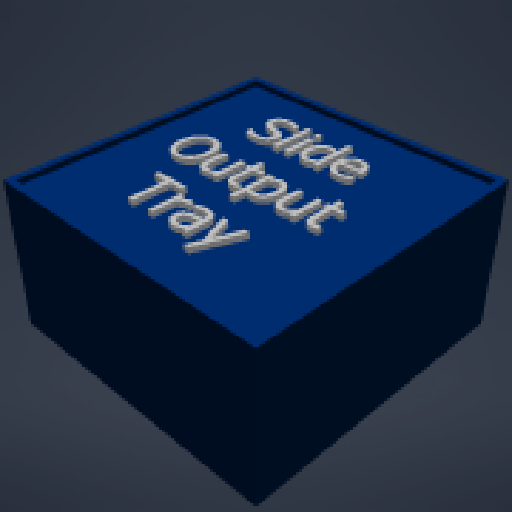
# Autodesk Inventor part: Slide Export Tray
Saved by Autodesk Inventor 2025.1 (Build 291241000, 241)
## iProperties
Created: 2024-10-31
Part Number: Slide Export Tray
Material: Generic
Document SubType Name: Modeling
Designer: jerem
Density: 1 g/cm^3
Appearance: Default
Author: jerem
Autodesk Inventor part; units mm, degrees
ref_plane "YZ Plane" through (0, 0, 0) normal (1, 0, 0) x (0, 1, 0)
ref_plane "XZ Plane" through (0, 0, 0) normal (0, 1, 0) x (-1, 0, 0)
ref_plane "XY Plane" through (0, 0, 0) normal (0, 0, 1) x (1, 0, 0)
sketch "Sketch1" plane through (0, 0, 0) normal (0, 1, 0) x (-1, 0, 0)
  line L0 (-50, 50) -> (50, 50)
  line L1 (50, 50) -> (50, -50)
  line L2 (50, -50) -> (-50, -50)
  line L3 (-50, -50) -> (-50, 50)
  line L4 (-50, 50) -> (50, -50) construction
  line L5 (50, 50) -> (-50, -50) construction
  line L6 (-47.5, 47.5) -> (47.5, 47.5)
  line L7 (47.5, 47.5) -> (47.5, -47.5)
  line L8 (47.5, -47.5) -> (-47.5, -47.5)
  line L9 (-47.5, -47.5) -> (-47.5, 47.5)
  line L10 (-47.5, 47.5) -> (47.5, -47.5) construction
  line L11 (47.5, 47.5) -> (-47.5, -47.5) construction
  point P0 (0, 0)
  dimension "d0" = 100
  dimension "d1" = 100
  dimension "d3" = 95
  constraints: 24 end point, 4 midpoint, 4 parallel, 2 horizontal, 2 perpendicular, 1 point on line
  measures "d0" distance of L1.end L2.end
  measures "d1" distance of L0.end L1.end
  measures "d3" distance of L7.end L8.end
extrude "Extrusion1" add sketch "Sketch1" along normal blind 50 contours L0 L1 L2 L3 | L6 L7 L8 L9
extrude "Extrusion2" add sketch "Sketch1" along normal blind 2 from surface at 50
sketch "Sketch2" plane through (0, 50, 0) normal (0, 1, 0) x (1, 0, 0)
  line L0 (-37.0883, 25.1556) -> (31.9282, 25.1556) construction
  line L1 (31.9282, 25.1556) -> (31.9282, -26.4456) construction
  line L2 (31.9282, -26.4456) -> (-37.0883, -26.4456) construction
  line L3 (-37.0883, -26.4456) -> (-37.0883, 25.1556) construction
  spline S0 degree 2 poles (-18.4674, 18.0229) (-20.0963, 18.0229) (-22.3815, 18.7036) (-23.3904, 19.1899) knots 0 0 0 1 2 2 2
  line L4 (-23.3904, 19.1899) -> (-23.3904, 21.6939)
  line L5 (-23.3904, 21.6939) -> (-23.2446, 21.6939)
  spline S1 degree 2 poles (-23.2446, 21.6939) (-22.26, 20.7701) (-19.7681, 19.749) (-18.6133, 19.749) knots 0 0 0 1 2 2 2
  spline S2 degree 2 poles (-18.6133, 19.749) (-16.9601, 19.749) (-15.2705, 21.1226) (-15.2705, 22.2531) knots 0 0 0 1 2 2 2
  spline S3 degree 2 poles (-15.2705, 22.2531) (-15.2705, 23.1526) (-16.1579, 24.2709) (-17.1181, 24.5505) knots 0 0 0 1 2 2 2
  spline S4 degree 2 poles (-17.1181, 24.5505) (-17.811, 24.745) (-18.9658, 25.0124) (-19.8288, 25.2312) knots 0 0 0 1 2 2 2
  spline S5 degree 2 poles (-19.8288, 25.2312) (-20.6068, 25.4378) (-21.8345, 26.0578) (-22.3086, 26.5561) knots 0 0 0 1 2 2 2
  spline S6 degree 2 poles (-22.3086, 26.5561) (-22.7705, 27.0545) (-23.281, 28.3916) (-23.281, 29.2668) knots 0 0 0 1 2 2 2
  spline S7 degree 2 poles (-23.281, 29.2668) (-23.281, 31.0902) (-20.4366, 33.5578) (-18.2365, 33.5578) knots 0 0 0 1 2 2 2
  spline S8 degree 2 poles (-18.2365, 33.5578) (-16.9723, 33.5578) (-14.7356, 33.0594) (-13.7754, 32.5853) knots 0 0 0 1 2 2 2
  line L6 (-13.7754, 32.5853) -> (-13.7754, 30.2028)
  line L7 (-13.7754, 30.2028) -> (-13.9212, 30.2028)
  spline S9 degree 2 poles (-13.9212, 30.2028) (-14.6384, 30.8592) (-16.875, 31.8317) (-18.1027, 31.8317) knots 0 0 0 1 2 2 2
  spline S10 degree 2 poles (-18.1027, 31.8317) (-19.4885, 31.8317) (-21.2024, 30.531) (-21.2024, 29.4735) knots 0 0 0 1 2 2 2
  spline S11 degree 2 poles (-21.2024, 29.4735) (-21.2024, 28.5253) (-20.1935, 27.3949) (-19.2454, 27.1396) knots 0 0 0 1 2 2 2
  spline S12 degree 2 poles (-19.2454, 27.1396) (-18.6133, 26.9694) (-16.7778, 26.5318) (-16.17, 26.3495) knots 0 0 0 1 2 2 2
  spline S13 degree 2 poles (-16.17, 26.3495) (-14.6262, 25.8754) (-13.1919, 23.967) (-13.1919, 22.5691) knots 0 0 0 1 2 2 2
  spline S14 degree 2 poles (-13.1919, 22.5691) (-13.1919, 21.6818) (-13.9091, 19.98) (-14.5533, 19.3843) knots 0 0 0 1 2 2 2
  spline S15 degree 2 poles (-14.5533, 19.3843) (-15.2705, 18.7279) (-17.0938, 18.0229) (-18.4674, 18.0229) knots 0 0 0 1 2 2 2
  line L8 (-9.375, 18.2903) -> (-11.2713, 18.2903)
  line L9 (-11.2713, 18.2903) -> (-11.2713, 33.9589)
  line L10 (-11.2713, 33.9589) -> (-9.375, 33.9589)
  line L11 (-9.375, 33.9589) -> (-9.375, 18.2903)
  line L12 (-4.6587, 18.2903) -> (-6.5549, 18.2903)
  line L13 (-6.5549, 18.2903) -> (-6.5549, 29.5464)
  line L14 (-6.5549, 29.5464) -> (-4.6587, 29.5464)
  line L15 (-4.6587, 29.5464) -> (-4.6587, 18.2903)
  line L16 (-4.525, 31.4184) -> (-6.6765, 31.4184)
  line L17 (-6.6765, 31.4184) -> (-6.6765, 33.3876)
  line L18 (-6.6765, 33.3876) -> (-4.525, 33.3876)
  line L19 (-4.525, 33.3876) -> (-4.525, 31.4184)
  line L20 (6.7797, 18.2903) -> (4.8835, 18.2903)
  line L21 (4.8835, 18.2903) -> (4.8835, 19.433)
  spline S16 degree 2 poles (4.8835, 19.433) (4.4459, 19.0683) (3.8016, 18.5821) (3.364, 18.3754) knots 0 0 0 1 2 2 2
  spline S17 degree 2 poles (3.364, 18.3754) (2.9629, 18.1809) (2.0998, 17.9743) (1.5285, 17.9743) knots 0 0 0 1 2 2 2
  spline S18 degree 2 poles (1.5285, 17.9743) (0.6047, 17.9743) (-0.9512, 18.7401) (-1.4982, 19.4816) knots 0 0 0 1 2 2 2
  spline S19 degree 2 poles (-1.4982, 19.4816) (-2.0452, 20.2231) (-2.653, 22.4111) (-2.653, 23.8333) knots 0 0 0 1 2 2 2
  spline S20 degree 2 poles (-2.653, 23.8333) (-2.653, 25.3163) (-1.8872, 27.48) (-1.2186, 28.2944) knots 0 0 0 1 2 2 2
  spline S21 degree 2 poles (-1.2186, 28.2944) (-0.5987, 29.0237) (1.1396, 29.8625) (2.0998, 29.8625) knots 0 0 0 1 2 2 2
  spline S22 degree 2 poles (2.0998, 29.8625) (2.9386, 29.8625) (4.1906, 29.4856) (4.8835, 29.0967) knots 0 0 0 1 2 2 2
  line L22 (4.8835, 29.0967) -> (4.8835, 33.9589)
  line L23 (4.8835, 33.9589) -> (6.7797, 33.9589)
  line L24 (6.7797, 33.9589) -> (6.7797, 18.2903)
  line L25 (4.8835, 21.0253) -> (4.8835, 27.5286)
  spline S23 degree 2 poles (4.8835, 27.5286) (4.1785, 27.8689) (3.0601, 28.1242) (2.4159, 28.1242) knots 0 0 0 1 2 2 2
  spline S24 degree 2 poles (2.4159, 28.1242) (0.9572, 28.1242) (-0.6959, 25.9362) (-0.6959, 23.8698) knots 0 0 0 1 2 2 2
  spline S25 degree 2 poles (-0.6959, 23.8698) (-0.6959, 21.8762) (0.5682, 19.7733) (1.9661, 19.7733) knots 0 0 0 1 2 2 2
  spline S26 degree 2 poles (1.9661, 19.7733) (2.7076, 19.7733) (4.2149, 20.454) (4.8835, 21.0253) knots 0 0 0 1 2 2 2
  spline S27 degree 2 poles (14.4135, 18.0351) (11.7149, 18.0351) (8.749, 21.0618) (8.749, 23.8576) knots 0 0 0 1 2 2 2
  spline S28 degree 2 poles (8.749, 23.8576) (8.749, 26.6048) (11.6298, 29.8625) (13.9515, 29.8625) knots 0 0 0 1 2 2 2
  spline S29 degree 2 poles (13.9515, 29.8625) (14.9969, 29.8625) (16.6136, 29.2547) (17.2092, 28.6104) knots 0 0 0 1 2 2 2
  spline S30 degree 2 poles (17.2092, 28.6104) (17.817, 27.9662) (18.4613, 26.1064) (18.4613, 24.7571) knots 0 0 0 1 2 2 2
  line L26 (18.4613, 24.7571) -> (18.4613, 23.7239)
  line L27 (18.4613, 23.7239) -> (10.6695, 23.7239)
  spline S31 degree 2 poles (10.6695, 23.7239) (10.6695, 21.7668) (12.6387, 19.6882) (14.3891, 19.6882) knots 0 0 0 1 2 2 2
  spline S32 degree 2 poles (14.3891, 19.6882) (15.0091, 19.6882) (16.2125, 19.9678) (16.6987, 20.1866) knots 0 0 0 1 2 2 2
  spline S33 degree 2 poles (16.6987, 20.1866) (17.2092, 20.4297) (17.9143, 20.8552) (18.1452, 21.0497) knots 0 0 0 1 2 2 2
  line L28 (18.1452, 21.0497) -> (18.2546, 21.0497)
  line L29 (18.2546, 21.0497) -> (18.2546, 18.9832)
  spline S34 degree 2 poles (18.2546, 18.9832) (17.9264, 18.8495) (16.9297, 18.4605) (16.5407, 18.3511) knots 0 0 0 1 2 2 2
  spline S35 degree 2 poles (16.5407, 18.3511) (15.9937, 18.1931) (15.0942, 18.0351) (14.4135, 18.0351) knots 0 0 0 1 2 2 2
  spline S36 degree 2 poles (16.6136, 25.1704) (16.5893, 25.9362) (16.2733, 27.0545) (15.9694, 27.4313) knots 0 0 0 1 2 2 2
  spline S37 degree 2 poles (15.9694, 27.4313) (15.6412, 27.8568) (14.6079, 28.3065) (13.8421, 28.3065) knots 0 0 0 1 2 2 2
  spline S38 degree 2 poles (13.8421, 28.3065) (13.0885, 28.3065) (12.031, 27.8568) (11.5934, 27.4192) knots 0 0 0 1 2 2 2
  spline S39 degree 2 poles (11.5934, 27.4192) (11.1679, 26.9694) (10.7303, 25.8876) (10.6695, 25.1704) knots 0 0 0 1 2 2 2
  line L30 (10.6695, 25.1704) -> (16.6136, 25.1704)
  spline S40 degree 2 poles (-21.8527, 6.8793) (-21.0019, 5.8825) (-20.0537, 2.9652) (-20.0537, 1.0932) knots 0 0 0 1 2 2 2
  spline S41 degree 2 poles (-20.0537, 1.0932) (-20.0537, -0.7301) (-20.9775, -3.6839) (-21.8527, -4.6807) knots 0 0 0 1 2 2 2
  spline S42 degree 2 poles (-21.8527, -4.6807) (-22.7766, -5.7261) (-25.2198, -6.7228) (-26.6907, -6.7228) knots 0 0 0 1 2 2 2
  spline S43 degree 2 poles (-26.6907, -6.7228) (-28.2101, -6.7228) (-30.6412, -5.6896) (-31.5286, -4.6807) knots 0 0 0 1 2 2 2
  spline S44 degree 2 poles (-31.5286, -4.6807) (-32.3916, -3.6839) (-33.3155, -0.7544) (-33.3155, 1.0932) knots 0 0 0 1 2 2 2
  spline S45 degree 2 poles (-33.3155, 1.0932) (-33.3155, 2.9774) (-32.3795, 5.8461) (-31.5164, 6.8793) knots 0 0 0 1 2 2 2
  spline S46 degree 2 poles (-31.5164, 6.8793) (-30.6412, 7.8761) (-28.198, 8.9093) (-26.6907, 8.9093) knots 0 0 0 1 2 2 2
  spline S47 degree 2 poles (-26.6907, 8.9093) (-25.1591, 8.9093) (-22.7036, 7.8396) (-21.8527, 6.8793) knots 0 0 0 1 2 2 2
  spline S48 degree 2 poles (-22.1323, 1.0932) (-22.1323, 2.5762) (-22.7766, 4.8736) (-23.36, 5.6273) knots 0 0 0 1 2 2 2
  spline S49 degree 2 poles (-23.36, 5.6273) (-23.9557, 6.4052) (-25.6331, 7.1832) (-26.6785, 7.1832) knots 0 0 0 1 2 2 2
  spline S50 degree 2 poles (-26.6785, 7.1832) (-27.7604, 7.1832) (-29.3892, 6.4295) (-30.0091, 5.6273) knots 0 0 0 1 2 2 2
  spline S51 degree 2 poles (-30.0091, 5.6273) (-30.6048, 4.8615) (-31.2369, 2.5519) (-31.2369, 1.0932) knots 0 0 0 1 2 2 2
  spline S52 degree 2 poles (-31.2369, 1.0932) (-31.2369, -1.8606) (-28.7571, -4.9967) (-26.6785, -4.9967) knots 0 0 0 1 2 2 2
  spline S53 degree 2 poles (-26.6785, -4.9967) (-24.5999, -4.9967) (-22.1323, -1.8606) (-22.1323, 1.0932) knots 0 0 0 1 2 2 2
  line L31 (-9.2596, -6.4068) -> (-11.1558, -6.4068)
  line L32 (-11.1558, -6.4068) -> (-11.1558, -5.1669)
  spline S54 degree 2 poles (-11.1558, -5.1669) (-12.031, -5.9327) (-13.5991, -6.7228) (-14.5715, -6.7228) knots 0 0 0 1 2 2 2
  spline S55 degree 2 poles (-14.5715, -6.7228) (-15.3009, -6.7228) (-16.6015, -6.2366) (-17.0756, -5.7139) knots 0 0 0 1 2 2 2
  spline S56 degree 2 poles (-17.0756, -5.7139) (-17.5618, -5.1912) (-18.0967, -3.5988) (-18.0967, -2.4562) knots 0 0 0 1 2 2 2
  line L33 (-18.0967, -2.4562) -> (-18.0967, 4.8493)
  line L34 (-18.0967, 4.8493) -> (-16.2004, 4.8493)
  line L35 (-16.2004, 4.8493) -> (-16.2004, -1.5688)
  spline S57 degree 2 poles (-16.2004, -1.5688) (-16.2004, -2.4684) (-16.0667, -3.6474) (-15.8357, -4.085) knots 0 0 0 1 2 2 2
  spline S58 degree 2 poles (-15.8357, -4.085) (-15.6048, -4.5226) (-14.8147, -4.9238) (-14.0732, -4.9238) knots 0 0 0 1 2 2 2
  spline S59 degree 2 poles (-14.0732, -4.9238) (-13.3803, -4.9238) (-11.8122, -4.1337) (-11.1558, -3.5624) knots 0 0 0 1 2 2 2
  line L36 (-11.1558, -3.5624) -> (-11.1558, 4.8493)
  line L37 (-11.1558, 4.8493) -> (-9.2596, 4.8493)
  line L38 (-9.2596, 4.8493) -> (-9.2596, -6.4068)
  spline S60 degree 2 poles (-3.1088, -6.6256) (-4.6526, -6.6256) (-6.3908, -4.863) (-6.3908, -2.9546) knots 0 0 0 1 2 2 2
  line L39 (-6.3908, -2.9546) -> (-6.3908, 3.2812)
  line L40 (-6.3908, 3.2812) -> (-7.6672, 3.2812)
  line L41 (-7.6672, 3.2812) -> (-7.6672, 4.8493)
  line L42 (-7.6672, 4.8493) -> (-6.3908, 4.8493)
  line L43 (-6.3908, 4.8493) -> (-6.3908, 8.0827)
  line L44 (-6.3908, 8.0827) -> (-4.4946, 8.0827)
  line L45 (-4.4946, 8.0827) -> (-4.4946, 4.8493)
  line L46 (-4.4946, 4.8493) -> (-1.0059, 4.8493)
  line L47 (-1.0059, 4.8493) -> (-1.0059, 3.2812)
  line L48 (-1.0059, 3.2812) -> (-4.4946, 3.2812)
  line L49 (-4.4946, 3.2812) -> (-4.4946, -2.0794)
  spline S61 degree 2 poles (-4.4946, -2.0794) (-4.4946, -2.9303) (-4.4338, -3.8662) (-4.2271, -4.2674) knots 0 0 0 1 2 2 2
  spline S62 degree 2 poles (-4.2271, -4.2674) (-4.057, -4.6199) (-3.2912, -4.9724) (-2.6348, -4.9724) knots 0 0 0 1 2 2 2
  spline S63 degree 2 poles (-2.6348, -4.9724) (-2.1728, -4.9724) (-1.3098, -4.6928) (-1.1153, -4.6077) knots 0 0 0 1 2 2 2
  line L50 (-1.1153, -4.6077) -> (-1.0059, -4.6077)
  line L51 (-1.0059, -4.6077) -> (-1.0059, -6.3095)
  spline S64 degree 2 poles (-1.0059, -6.3095) (-1.5408, -6.4554) (-2.6348, -6.6256) (-3.1088, -6.6256) knots 0 0 0 1 2 2 2
  spline S65 degree 2 poles (9.8247, -0.4748) (9.8247, -3.2949) (7.1383, -6.6256) (5.084, -6.6256) knots 0 0 0 1 2 2 2
  spline S66 degree 2 poles (5.084, -6.6256) (4.2453, -6.6256) (2.9568, -6.2366) (2.2883, -5.8355) knots 0 0 0 1 2 2 2
  line L52 (2.2883, -5.8355) -> (2.2883, -10.5518)
  line L53 (2.2883, -10.5518) -> (0.392, -10.5518)
  line L54 (0.392, -10.5518) -> (0.392, 4.8493)
  line L55 (0.392, 4.8493) -> (2.2883, 4.8493)
  line L56 (2.2883, 4.8493) -> (2.2883, 3.6702)
  spline S67 degree 2 poles (2.2883, 3.6702) (2.9933, 4.3145) (4.7194, 5.1654) (5.7283, 5.1654) knots 0 0 0 1 2 2 2
  spline S68 degree 2 poles (5.7283, 5.1654) (7.661, 5.1654) (9.8247, 2.1021) (9.8247, -0.4748) knots 0 0 0 1 2 2 2
  spline S69 degree 2 poles (7.8677, -0.6936) (7.8677, 1.2391) (6.64, 3.3663) (5.2664, 3.3663) knots 0 0 0 1 2 2 2
  spline S70 degree 2 poles (5.2664, 3.3663) (4.4641, 3.3663) (2.9568, 2.6492) (2.2883, 2.09) knots 0 0 0 1 2 2 2
  line L57 (2.2883, 2.09) -> (2.2883, -4.3038)
  spline S71 degree 2 poles (2.2883, -4.3038) (3.0297, -4.6564) (4.0873, -4.9238) (4.768, -4.9238) knots 0 0 0 1 2 2 2
  spline S72 degree 2 poles (4.768, -4.9238) (6.2388, -4.9238) (7.8677, -2.7601) (7.8677, -0.6936) knots 0 0 0 1 2 2 2
  line L58 (20.546, -6.4068) -> (18.6497, -6.4068)
  line L59 (18.6497, -6.4068) -> (18.6497, -5.1669)
  spline S73 degree 2 poles (18.6497, -5.1669) (17.7745, -5.9327) (16.2064, -6.7228) (15.234, -6.7228) knots 0 0 0 1 2 2 2
  spline S74 degree 2 poles (15.234, -6.7228) (14.5046, -6.7228) (13.204, -6.2366) (12.7299, -5.7139) knots 0 0 0 1 2 2 2
  spline S75 degree 2 poles (12.7299, -5.7139) (12.2437, -5.1912) (11.7088, -3.5988) (11.7088, -2.4562) knots 0 0 0 1 2 2 2
  line L60 (11.7088, -2.4562) -> (11.7088, 4.8493)
  line L61 (11.7088, 4.8493) -> (13.6051, 4.8493)
  line L62 (13.6051, 4.8493) -> (13.6051, -1.5688)
  spline S76 degree 2 poles (13.6051, -1.5688) (13.6051, -2.4684) (13.7388, -3.6474) (13.9698, -4.085) knots 0 0 0 1 2 2 2
  spline S77 degree 2 poles (13.9698, -4.085) (14.2007, -4.5226) (14.9909, -4.9238) (15.7323, -4.9238) knots 0 0 0 1 2 2 2
  spline S78 degree 2 poles (15.7323, -4.9238) (16.4252, -4.9238) (17.9933, -4.1337) (18.6497, -3.5624) knots 0 0 0 1 2 2 2
  line L63 (18.6497, -3.5624) -> (18.6497, 4.8493)
  line L64 (18.6497, 4.8493) -> (20.546, 4.8493)
  line L65 (20.546, 4.8493) -> (20.546, -6.4068)
  spline S79 degree 2 poles (26.6967, -6.6256) (25.1529, -6.6256) (23.4147, -4.863) (23.4147, -2.9546) knots 0 0 0 1 2 2 2
  line L66 (23.4147, -2.9546) -> (23.4147, 3.2812)
  line L67 (23.4147, 3.2812) -> (22.1383, 3.2812)
  line L68 (22.1383, 3.2812) -> (22.1383, 4.8493)
  line L69 (22.1383, 4.8493) -> (23.4147, 4.8493)
  line L70 (23.4147, 4.8493) -> (23.4147, 8.0827)
  line L71 (23.4147, 8.0827) -> (25.3109, 8.0827)
  line L72 (25.3109, 8.0827) -> (25.3109, 4.8493)
  line L73 (25.3109, 4.8493) -> (28.7996, 4.8493)
  line L74 (28.7996, 4.8493) -> (28.7996, 3.2812)
  line L75 (28.7996, 3.2812) -> (25.3109, 3.2812)
  line L76 (25.3109, 3.2812) -> (25.3109, -2.0794)
  spline S80 degree 2 poles (25.3109, -2.0794) (25.3109, -2.9303) (25.3717, -3.8662) (25.5784, -4.2674) knots 0 0 0 1 2 2 2
  spline S81 degree 2 poles (25.5784, -4.2674) (25.7485, -4.6199) (26.5144, -4.9724) (27.1708, -4.9724) knots 0 0 0 1 2 2 2
  spline S82 degree 2 poles (27.1708, -4.9724) (27.6327, -4.9724) (28.4957, -4.6928) (28.6902, -4.6077) knots 0 0 0 1 2 2 2
  line L77 (28.6902, -4.6077) -> (28.7996, -4.6077)
  line L78 (28.7996, -4.6077) -> (28.7996, -6.3095)
  spline S83 degree 2 poles (28.7996, -6.3095) (28.2648, -6.4554) (27.1708, -6.6256) (26.6967, -6.6256) knots 0 0 0 1 2 2 2
  line L79 (-17.8536, -31.1039) -> (-17.8536, -17.8786)
  line L80 (-17.8536, -17.8786) -> (-22.886, -17.8786)
  line L81 (-22.886, -17.8786) -> (-22.886, -16.1039)
  line L82 (-22.886, -16.1039) -> (-10.8276, -16.1039)
  line L83 (-10.8276, -16.1039) -> (-10.8276, -17.8786)
  line L84 (-10.8276, -17.8786) -> (-15.86, -17.8786)
  line L85 (-15.86, -17.8786) -> (-15.86, -31.1039)
  line L86 (-15.86, -31.1039) -> (-17.8536, -31.1039)
  line L87 (-3.4856, -21.8778) -> (-3.5829, -21.8778)
  spline S84 degree 2 poles (-3.5829, -21.8778) (-3.8017, -21.817) (-4.2758, -21.7927) (-4.604, -21.7927) knots 0 0 0 1 2 2 2
  spline S85 degree 2 poles (-4.604, -21.7927) (-5.3698, -21.7927) (-6.8771, -22.4612) (-7.5578, -23.1176) knots 0 0 0 1 2 2 2
  line L88 (-7.5578, -23.1176) -> (-7.5578, -31.1039)
  line L89 (-7.5578, -31.1039) -> (-9.454, -31.1039)
  line L90 (-9.454, -31.1039) -> (-9.454, -19.8478)
  line L91 (-9.454, -19.8478) -> (-7.5578, -19.8478)
  line L92 (-7.5578, -19.8478) -> (-7.5578, -21.5253)
  spline S86 degree 2 poles (-7.5578, -21.5253) (-6.5245, -20.6014) (-4.9808, -19.8478) (-4.2515, -19.8478) knots 0 0 0 1 2 2 2
  spline S87 degree 2 poles (-4.2515, -19.8478) (-3.9597, -19.8478) (-3.668, -19.8721) (-3.4856, -19.9086) knots 0 0 0 1 2 2 2
  line L93 (-3.4856, -19.9086) -> (-3.4856, -21.8778)
  spline S88 degree 2 poles (4.2575, -29.9126) (4.0265, -30.0828) (3.2485, -30.6906) (2.8839, -30.8729) knots 0 0 0 1 2 2 2
  spline S89 degree 2 poles (2.8839, -30.8729) (2.3855, -31.1403) (1.4495, -31.4199) (0.5986, -31.4199) knots 0 0 0 1 2 2 2
  spline S90 degree 2 poles (0.5986, -31.4199) (-0.0942, -31.4199) (-1.3463, -30.8972) (-1.8203, -30.4232) knots 0 0 0 1 2 2 2
  spline S91 degree 2 poles (-1.8203, -30.4232) (-2.2701, -29.9612) (-2.8171, -28.5998) (-2.8171, -27.8462) knots 0 0 0 1 2 2 2
  spline S92 degree 2 poles (-2.8171, -27.8462) (-2.8171, -26.6792) (-1.8325, -25.0261) (-0.7628, -24.552) knots 0 0 0 1 2 2 2
  spline S93 degree 2 poles (-0.7628, -24.552) (0.1853, -24.1144) (2.7623, -23.7862) (4.2575, -23.7011) knots 0 0 0 1 2 2 2
  line L94 (4.2575, -23.7011) -> (4.2575, -23.3364)
  spline S94 degree 2 poles (4.2575, -23.3364) (4.2575, -22.68) (3.8563, -21.8656) (3.4917, -21.6347) knots 0 0 0 1 2 2 2
  spline S95 degree 2 poles (3.4917, -21.6347) (3.127, -21.4037) (2.0816, -21.2578) (1.5225, -21.2578) knots 0 0 0 1 2 2 2
  spline S96 degree 2 poles (1.5225, -21.2578) (0.8661, -21.2578) (-0.9087, -21.6468) (-1.796, -22.0236) knots 0 0 0 1 2 2 2
  line L95 (-1.796, -22.0236) -> (-1.9054, -22.0236)
  line L96 (-1.9054, -22.0236) -> (-1.9054, -20.0909)
  spline S97 degree 2 poles (-1.9054, -20.0909) (-1.3827, -19.945) (0.5743, -19.5804) (1.5346, -19.5804) knots 0 0 0 1 2 2 2
  spline S98 degree 2 poles (1.5346, -19.5804) (2.7015, -19.5804) (4.2939, -19.945) (4.926, -20.4191) knots 0 0 0 1 2 2 2
  spline S99 degree 2 poles (4.926, -20.4191) (5.546, -20.881) (6.1537, -22.3518) (6.1537, -23.4094) knots 0 0 0 1 2 2 2
  line L97 (6.1537, -23.4094) -> (6.1537, -31.1039)
  line L98 (6.1537, -31.1039) -> (4.2575, -31.1039)
  line L99 (4.2575, -31.1039) -> (4.2575, -29.9126)
  line L100 (4.2575, -28.3324) -> (4.2575, -25.2084)
  spline S100 degree 2 poles (4.2575, -25.2084) (3.5767, -25.2692) (1.5225, -25.4758) (0.8782, -25.6703) knots 0 0 0 1 2 2 2
  spline S101 degree 2 poles (0.8782, -25.6703) (0.1246, -25.9013) (-0.86, -26.8616) (-0.86, -27.7125) knots 0 0 0 1 2 2 2
  spline S102 degree 2 poles (-0.86, -27.7125) (-0.86, -28.6849) (0.234, -29.6695) (1.2793, -29.6695) knots 0 0 0 1 2 2 2
  spline S103 degree 2 poles (1.2793, -29.6695) (2.1667, -29.6695) (3.6254, -28.9037) (4.2575, -28.3324) knots 0 0 0 1 2 2 2
  line L101 (17.6529, -19.8478) -> (11.5994, -35.2489)
  line L102 (11.5994, -35.2489) -> (9.5695, -35.2489)
  line L103 (9.5695, -35.2489) -> (11.5873, -30.5569)
  line L104 (11.5873, -30.5569) -> (7.503, -19.8478)
  line L105 (7.503, -19.8478) -> (9.5451, -19.8478)
  line L106 (9.5451, -19.8478) -> (12.6205, -28.1865)
  line L107 (12.6205, -28.1865) -> (15.6837, -19.8478)
  line L108 (15.6837, -19.8478) -> (17.6529, -19.8478)
  point P0 (0, 0)
  constraints: 2 other
extrude "Extrusion3" add sketch "Sketch2" along normal blind 2
body "Solid1"
